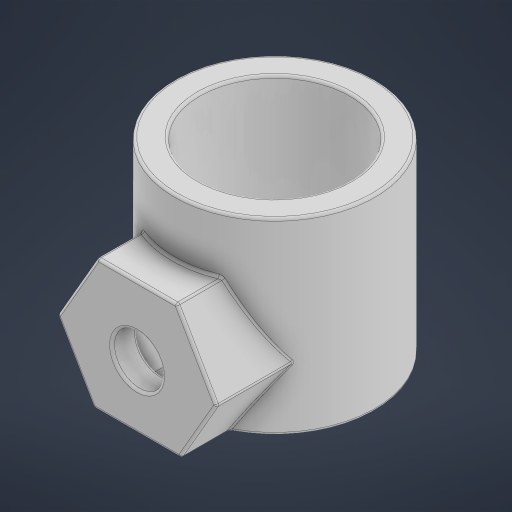
# Autodesk Inventor part: nut_holder
Saved by Autodesk Inventor 2023 (Build 270158000, 158)
## iProperties
Created: 2022-05-26
Part Number: nut_holder
Material: Generic
Document SubType Name: Modeling
Designer: Norbert Ligas
Density: 1 g/cm^3
Appearance: Default
Author: Norbert Ligas
Autodesk Inventor part; units mm, degrees
ref_plane "YZ Plane" through (0, 0, 0) normal (1, 0, 0) x (0, 1, 0)
ref_plane "XZ Plane" through (0, 0, 0) normal (0, 1, 0) x (-1, 0, 0)
ref_plane "XY Plane" through (0, 0, 0) normal (0, 0, 1) x (1, 0, 0)
sketch "Sketch1" plane through (0, 0, 0) normal (0, 1, 0) x (-1, 0, 0)
  circle A0 centre (0, 0) radius 8
  circle A1 centre (0, 0) radius 6
  dimension "d1" = 12
  dimension "d3" = 2
  constraints: 2 centre point, 2 coincident
  measures "d1" diameter of A1
  measures "d3" radial gap between concentric circles of A0 A1
extrude "Extrusion1" add sketch "Sketch1" along normal blind 15
sketch "Sketch2" plane through (0, 0, 0) normal (0, 0, 1) x (1, 0, 0)
  line L0 (8, 15) -> (-8, 15) projected
  line L1 (8, 0) -> (-8, 0) projected
  line L2 (8, 15) -> (-8, 15) projected
  line L3 (-8, 0) -> (-8, 15) projected
  line L4 (8, 0) -> (-8, 0) projected
  line L5 (8, 0) -> (8, 15) projected
  line L6 (0, -3) -> (0, 18) projected
  line L7 (2.0207, 8.5) -> (4.0415, 5)
  line L8 (4.0415, 5) -> (2.0207, 1.5)
  line L9 (2.0207, 1.5) -> (-2.0207, 1.5)
  line L10 (-2.0207, 1.5) -> (-4.0415, 5)
  line L11 (-4.0415, 5) -> (-2.0207, 8.5)
  line L12 (-2.0207, 8.5) -> (2.0207, 8.5)
  line L13 (6.3509, 5) -> (3.4641, 0)
  line L14 (3.4641, 0) -> (-3.4641, 0)
  line L15 (-3.4641, 0) -> (-6.3509, 5)
  line L16 (-6.3509, 5) -> (-3.1754, 10.5)
  line L17 (-3.1754, 10.5) -> (3.1754, 10.5)
  line L18 (3.1754, 10.5) -> (6.3509, 5)
  point P0 (0, 0)
  point P1 (0, 5)
  point P2 (0, 8.5)
  point P3 (0, 5)
  dimension "d6" = 10
  dimension "d9" = 7
  dimension "d11" = 2
  constraints: 24 end point, 4 point on line, 2 parallel, 1 coincident, 1 midpoint, 21 other
  measures "d6" distance from line of L0 point (0, 5)
  measures "d9" distance between parallel lines of L9 L12
  measures "d11" distance between parallel lines of L17 L12
extrude "Extrusion2" add sketch "Sketch2" along normal blind 11 contours L17 L18 L13 L1 L6 L9 L8 L7 L12 | L6 L12 L11 L10 L9 L1 L15 L16 L17 | L12 L7 L8 L9 L6 | L6 L9 L10 L11 L12
extrude "Extrusion3" cut sketch "Sketch2" along normal blind 9 contours L12 L7 L8 L9 L6 | L6 L9 L10 L11 L12
extrude "Extrusion4" cut sketch "Sketch1" along normal blind 15 contours A1
sketch "Sketch3" plane through (0, 0, 11) normal (0, 0, 1) x (1, 0, 0)
  line L0 (3.4641, 0) -> (6.3509, 5) projected
  line L1 (6.3509, 5) -> (3.1754, 10.5) projected
  line L2 (3.1754, 10.5) -> (-3.1754, 10.5) projected
  line L3 (-3.1754, 10.5) -> (-6.3509, 5) projected
  line L4 (-6.3509, 5) -> (-3.4641, 0) projected
  line L5 (-3.4641, 0) -> (3.4641, 0) projected
  line L6 (0, -3) -> (0, 18) projected
  line L7 (6.3509, 5) -> (-6.3509, 5) construction
  line L8 (6, 15) -> (6, 0) projected
  line L9 (6, 15) -> (6, 0) construction
  line L10 (6, 15) -> (6, 0) projected
  line L11 (6, 15) -> (6, 0) projected
  line L12 (6, 15) -> (6, 0) projected
  circle A0 centre (0, 5) radius 2
  point P0 (0, 0)
  dimension "d18" = 4
  constraints: 2 end point, 1 centre point, 1 coincident, 1 horizontal, 1 midpoint, 1 point on line, 2 other
  measures "d18" diameter of A0
extrude "Extrusion5" cut sketch "Sketch3" against normal blind 2 contours A0 L6 | L6 A0
fillet "Fillet1" radius 0.2 30 edges at (0, 10.5, 11) (3.1754, 10.5, 9.1714) (0, 10.5, 8) (4.9216, 7.4755, 6.3069) (4.7631, 7.75, 11) (6.3509, 5, 7.9324) (5.0457, 2.7395, 6.2081) (4.9075, 2.5, 11) (3.4641, 0, 9.1056) (-6.7717, 0, 4.2595) (4.2595, 0, -6.7717) (6, 0, 0) (-3.4641, 0, 9.1056) (0, 0, 11) (-2, 5, 11) (-2, 5, 9) (-4.9075, 2.5, 11) (-4.7631, 7.75, 11) (-4.9216, 7.4755, 6.3069) (-5.0457, 2.7395, 6.2081) (-6.3509, 5, 7.9324) (-3.1754, 10.5, 9.1714) (8, 15, 0) (6, 15, 0) (0, 8.5, 6) (3.0913, 6.6456, 5.1423) (-3.0913, 6.6456, 5.1423) (-3.0913, 3.3544, 5.1423) (0, 1.5, 6) (3.0913, 3.3544, 5.1423)
equation "\"d1\" = inside_diameter"
equation "\"d3\" = thickness"
equation "\"d4\" = length"
equation "\"d6\" = hole_to_edge"
equation "\"d9\" = nut_width"
equation "\"d11\" = thickness"
equation "\"d12\" = bay_outer_edge_to_center"
equation "\"d14\" = bay_inner_distance_to_center"
equation "\"d16\" = length"
equation "\"d18\" = hole_diameter"
equation "\"d19\" = thickness"
equation "\"thickness\" = 2"
equation "\"length\" = 15"
equation "\"hole_to_edge\" = 10"
equation "\"nut_width\" = 7"
equation "\"nut_bay_outer_height\" = nut_height + thickness"
equation "\"nut_height\" = 3"
equation "\"inside_diameter\" = 12"
equation "\"bay_outer_edge_to_center\" = nut_bay_outer_height + 0.5 * inside_diameter"
equation "\"bay_inner_distance_to_center\" = nut_height + 0.5 * inside_diameter"
equation "\"hole_diameter\" = 4"
body "Solid1"
